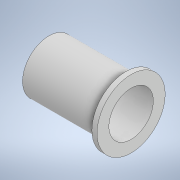
# Autodesk Inventor part: Sunroof Drain Tube Insert
Saved by Autodesk Inventor 2021 (Build 250183000, 183)
## iProperties
Created: 2021-10-24
Part Number: Sunroof Drain Tube Insert
Material: Generic
Document SubType Name: Modeling
Designer: Andrew
Density: 1 g/cm^3
Appearance: Default
Author: Andrew
Autodesk Inventor part; units mm, degrees
ref_plane "YZ Plane" through (0, 0, 0) normal (1, 0, 0) x (0, 1, 0)
ref_plane "XZ Plane" through (0, 0, 0) normal (0, 1, 0) x (-1, 0, 0)
ref_plane "XY Plane" through (0, 0, 0) normal (0, 0, 1) x (1, 0, 0)
sketch "Sketch1" plane through (0, 0, 0) normal (0, 0, 1) x (1, 0, 0)
  line L0 (0, 5.125) -> (15, 5.125)
  line L1 (15, 5.125) -> (15, 6.625)
  line L2 (15, 6.625) -> (0, 6.625)
  line L3 (0, 6.625) -> (0, 5.125)
  line L4 (0, 5.125) -> (15, 5.125)
  line L5 (15, 5.125) -> (15, 6.625)
  line L6 (15, 6.625) -> (16, 6.625)
  line L7 (16, 6.625) -> (16, 4.325)
  line L8 (16, 4.325) -> (0, 4.325)
  line L9 (0, 4.325) -> (0, 5.125)
  line L10 (-3.2, 0) -> (19.2, 0) projected
  point P0 (0, 0)
  dimension "d0" = 1.5
  dimension "d1" = 15
  dimension "d2" = 6.625
  dimension "d3" = 0.8
  dimension "d4" = 1
  constraints: 20 end point, 7 perpendicular, 5 point on line, 2 collinear, 2 horizontal
  measures "d0" distance between parallel lines of L0 L2
  measures "d1" distance of L1.end L2.end
  measures "d2" distance from line of point (0, 0) L2
  measures "d3" distance of L8.end L4.start
  measures "d4" distance between parallel lines of L1 L7
revolve "Revolution1" add sketch "Sketch1" angle 360 about axis through (-10, 0, 0) along (1, 0, 0) contours L0 L1 L6 L7 L8 L9
body "Solid1"
